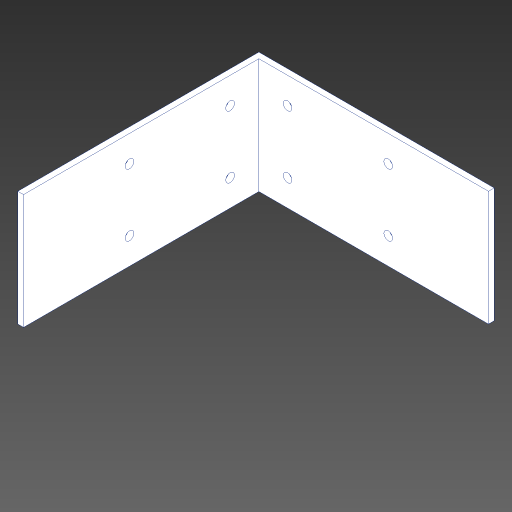
# Autodesk Inventor part: BDVBS_002_Brachet 2
Saved by Autodesk Inventor 2024 (Build 280153000, 153)
## iProperties
Created: 2024-08-05
Part Number: BDVBS_002_Brachet 2
Material: Aluminum 6061
Document SubType Name: Modeling
Designer: sarav
Density: 2.7 g/cm^3
Appearance: Aluminum - Flat
Author: sarav
Autodesk Inventor part; units mm, degrees
ref_plane "YZ Plane" through (0, 0, 0) normal (1, 0, 0) x (0, 1, 0)
ref_plane "XZ Plane" through (0, 0, 0) normal (0, 1, 0) x (-1, 0, 0)
ref_plane "XY Plane" through (0, 0, 0) normal (0, 0, 1) x (1, 0, 0)
sketch "Sketch1" plane through (0, 0, 0) normal (0, 0, 1) x (1, 0, 0)
  line L0 (0, 0) -> (103.9622, 0)
  line L1 (103.9622, 0) -> (103.9622, 50.8)
  line L2 (103.9622, 50.8) -> (0, 50.8)
  line L3 (0, 50.8) -> (0, 0)
  line L4 (0, 50.8) -> (103.9622, 50.8)
  line L5 (103.9622, 50.8) -> (103.9622, 42.9936)
  line L6 (0, 42.9936) -> (0, 50.8)
  dimension "d4" = 103.9622
  dimension "d5" = 50.8
  constraints: 14 end point, 3 parallel, 2 horizontal, 2 perpendicular, 1 point on line
  measures "d4" distance of L2.end L1.end
  measures "d5" distance of L1.end L0.end
extrude "Extrusion1" add sketch "Sketch1" along normal blind 2.54
sketch "Sketch6" plane through (0, 0, 2.54) normal (0, 0, 1) x (1, 0, 0)
  line L0 (103.9622, 0) -> (103.9622, 50.8) projected
  line L1 (103.9622, 50.8) -> (0, 50.8) projected
  line L2 (0, 50.8) -> (0, 0) projected
  line L3 (0, 0) -> (103.9622, 0) projected
  line L4 (0, 0) -> (2.54, 0)
  line L5 (2.54, 0) -> (2.54, 50.8)
  line L6 (2.54, 50.8) -> (0, 50.8)
  line L7 (0, 50.8) -> (0, 0)
  dimension "d23" = 2.54
  dimension "d24" = 50.8
  constraints: 8 end point, 2 parallel, 1 horizontal, 1 perpendicular
  measures "d23" distance of L6.end L5.end
  measures "d24" distance of L5.end L4.end
extrude "Extrusion5" add sketch "Sketch6" along normal blind 103.9622 contours L3 L2 L1 L5
sketch "Sketch7" plane through (2.54, 0, 2.54) normal (1, 0, 0) x (0, 0, -1)
  line L0 (0, 50.8) -> (0, 0) projected
  line L1 (0, 50.8) -> (-103.9622, 50.8) projected
  line L2 (-103.9622, 0) -> (-103.9622, 50.8) projected
  line L3 (0, 0) -> (-103.9622, 0) projected
  line L4 (2.54, 0) -> (2.54, 50.8) projected
  line L5 (2.54, 50.8) -> (0, 50.8) projected
  line L6 (0, 0) -> (0, 50.8) projected
  line L7 (2.54, 0) -> (0, 0) projected
  line L8 (0, 50.8) -> (0, 0) projected
  line L9 (0, 50.8) -> (-103.9622, 50.8) projected
  line L10 (-103.9622, 0) -> (-103.9622, 50.8) projected
  line L11 (0, 0) -> (-103.9622, 0) projected
  circle A0 centre (-12.7, 39.1541) radius 1.905
  circle A1 centre (-12.7, 11.6459) radius 1.905
  circle A2 centre (-57.15, 39.1541) radius 1.905
  circle A3 centre (-57.15, 11.6459) radius 1.905
  dimension "d27" = 3.81
  dimension "d28" = 11.6459
  dimension "d29" = 12.7
  dimension "d30" = 3.81
  dimension "d31" = 11.6459
  dimension "d32" = 3.81
  dimension "d33" = 3.81
  dimension "d34" = 44.45
  dimension "d35" = 44.45
  dimension "d36" = 11.6459
  dimension "d37" = 12.7
  dimension "d38" = 11.6459
  constraints: 4 centre point
  measures "d27" diameter of A0
  measures "d28" distance from line of A0.centre L1
  measures "d29" distance from line of L0 A0.centre
  measures "d30" diameter of A1
  measures "d31" distance from line of L3 A1.centre
  measures "d32" diameter of A2
  measures "d33" diameter of A3
  measures "d34" distance of A0.centre A2.centre
  measures "d35" distance of A3.centre A1.centre
  measures "d36" distance from line of L9 A2.centre
  measures "d37" distance from line of L0 A1.centre
  measures "d38" distance from line of L3 A3.centre
extrude "Extrusion6" cut sketch "Sketch7" against normal through all contours A0 | A1 | A2 | A3
sketch "Sketch8" plane through (0, 0, 2.54) normal (0, 0, 1) x (1, 0, 0)
  circle A0 centre (15.24, 39.1541) radius 1.905
  circle A1 centre (15.24, 11.6459) radius 1.905
  circle A2 centre (59.69, 39.1541) radius 1.905
  circle A3 centre (59.69, 11.6459) radius 1.905
  line L0 (103.9622, 50.8) -> (2.54, 50.8) projected
  line L1 (2.54, 0) -> (103.9622, 0) projected
  line L2 (2.54, 0) -> (2.54, 50.8) projected
  point P0 (0, 0)
  dimension "d41" = 3.81
  dimension "d42" = 3.81
  dimension "d43" = 3.81
  dimension "d44" = 3.81
  dimension "d45" = 11.6459
  dimension "d46" = 11.6459
  dimension "d47" = 11.6459
  dimension "d48" = 11.6459
  dimension "d49" = 12.7
  dimension "d50" = 12.7
  dimension "d51" = 44.45
  dimension "d52" = 44.45
  constraints: 4 centre point
  measures "d41" diameter of A0
  measures "d42" diameter of A1
  measures "d43" diameter of A2
  measures "d44" diameter of A3
  measures "d45" distance from line of L0 A0.centre
  measures "d46" distance from line of L0 A2.centre
  measures "d47" distance from line of L1 A1.centre
  measures "d48" distance from line of L1 A3.centre
  measures "d49" distance from line of L2 A0.centre
  measures "d50" distance from line of L2 A1.centre
  measures "d51" distance of A2.centre A0.centre
  measures "d52" distance of A1.centre A3.centre
extrude "Extrusion7" cut sketch "Sketch8" against normal through all
body "Solid1"
